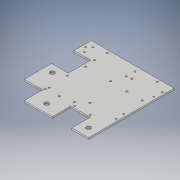
# Autodesk Inventor part: КВ33.044.002 - Дно платы
Saved by Autodesk Inventor 2019 (Build 230136000, 136)
## iProperties
Created: 2019-10-30
Part Number: КВ33.044.002 - Дно платы
Material: Типовые
Document SubType Name: Modeling
Designer: Петров Иван
Density: 1 g/cm^3
Appearance: По умолчанию
Mass: 56.5933 g
Surface Area: 408.613 cm^2
Volume: 56.5933 cm^3
Author: Петров Иван
Autodesk Inventor part; units mm, degrees
ref_plane "YZ Plane" through (0, 0, 0) normal (1, 0, 0) x (0, 1, 0)
ref_plane "XZ Plane" through (0, 0, 0) normal (0, 1, 0) x (-1, 0, 0)
ref_plane "XY Plane" through (0, 0, 0) normal (0, 0, 1) x (1, 0, 0)
sketch "Эскиз1" plane through (0, 0, 0) normal (0, 1, 0) x (-1, 0, 0)
  line L0 (-25, 35) -> (25, 35)
  line L1 (25, 35) -> (25, -35)
  line L2 (25, -35) -> (-25, -35)
  line L3 (-25, -35) -> (-25, 35)
  line L4 (-22.5, 32.5) -> (22.5, 32.5)
  line L5 (22.5, 31.5) -> (22.5, -31)
  line L6 (22.5, -32.5) -> (-22.5, -32.5)
  circle A0 centre (22.5, 32.5) radius 1.5
  circle A1 centre (22.5, -32.5) radius 1.5
  circle A2 centre (-22.5, -32.5) radius 1.5
  circle A3 centre (-22.5, 32.5) radius 1.5
  line L7 (-25, 35) -> (-23.7767, 33.2874) construction
  line L8 (-22.5, -31) -> (-22.5, 31)
  line L9 (23.7767, -33.2874) -> (25, -35) construction
  line L10 (25, -30.9585) -> (25, 35)
  line L11 (25, 35) -> (-25, 35)
  line L12 (25, 35) -> (25, -35)
  point P0 (0, 0)
  dimension "d6" = 3
  dimension "d0" = 50
  dimension "d2" = 45
  dimension "d4" = 3
  dimension "d5" = 3
  dimension "d7" = 3
  constraints: 26 end point, 4 coincident, 4 parallel, 4 point on circle, 3 centre point, 3 horizontal, 2 perpendicular, 2 point on line, 1 vertical alignment, 2 other
  measures "d0" distance of L1.end L2.end
  measures "d2" distance of L6.start L6.end
  measures "d4" diameter of A0
  measures "d5" diameter of A1
  measures "d7" diameter of A3
extrude "Выдавливание1" add sketch "Эскиз1" along normal blind 3 contours L0 L1 L2 L3 | L4 A0 L5 A1 L6 A2 L8 A3
sketch "Эскиз2" plane through (0, 3, 0) normal (0, 1, 0) x (1, 0, 0)
  line L0 (-25, -35) -> (25, -35) projected
  line L1 (-25, -35) -> (-28, -35)
  line L2 (-28, -35) -> (-28, 35)
  line L3 (-28, 35) -> (-25, 35)
  line L4 (-25, 35) -> (-25, -35)
  line L5 (-28, -35) -> (-58, -35)
  line L6 (-58, -35) -> (-58, 35)
  line L7 (-58, 35) -> (-28, 35)
  line L8 (-28, 35) -> (-28, -35)
  line L9 (-25, -35) -> (25, -35)
  line L10 (25, -35) -> (25, -38)
  line L11 (25, -38) -> (-25, -38)
  line L12 (-25, -38) -> (-25, -35)
  line L13 (-25, -38) -> (25, -38)
  line L14 (25, -38) -> (25, -68)
  line L15 (25, -68) -> (-25, -68)
  line L16 (-25, -68) -> (-25, -38)
  line L17 (-25, -68) -> (0, -68)
  line L18 (0, -53) -> (-25, -53)
  line L19 (-25, -53) -> (-25, -68)
  circle A0 centre (0, -53) radius 4
  line L20 (-58, 0) -> (-43, 0)
  circle A1 centre (-43, 0) radius 4
  point P0 (0, 0)
  dimension "d18" = 3
  dimension "d19" = 70
  dimension "d20" = 30
  dimension "d21" = 70
  dimension "d22" = 50
  dimension "d23" = 3
  dimension "d24" = 50
  dimension "d25" = 30
  dimension "d26" = 25
  dimension "d27" = 15
  dimension "d28" = 8
  dimension "d29" = 15
  dimension "d30" = 8
  constraints: 40 end point, 9 parallel, 6 horizontal, 4 perpendicular, 2 centre point, 2 coincident, 1 midpoint
  measures "d18" distance of L2.end L3.end
  measures "d19" distance of L1.end L2.end
  measures "d20" distance of L6.end L7.end
  measures "d21" distance of L5.end L6.end
  measures "d22" distance of L10.end L11.end
  measures "d23" distance of L9.end L10.end
  measures "d24" distance of L14.end L15.end
  measures "d25" distance of L13.end L14.end
  measures "d26" distance of L18.end L18.start
  measures "d27" distance of L18.start L17.end
  measures "d28" diameter of A0
  measures "d29" distance of L20.start L20.end
  measures "d30" diameter of A1
extrude "Выдавливание2" add sketch "Эскиз2" against normal blind 3
sketch "Эскиз3" plane through (0, 3, 0) normal (0, 1, 0) x (1, 0, 0)
  line L0 (-58, -35) -> (-25, -35) projected
  line L1 (-25, -35) -> (25, -35)
  line L2 (25, 35) -> (25, -68) projected
  line L3 (25, -35) -> (75, -35)
  line L4 (75, -35) -> (75, 35)
  line L5 (75, 35) -> (25, 35)
  line L6 (25, 35) -> (25, -35)
  point P0 (0, 0)
  dimension "d33" = 50
  constraints: 10 end point, 2 horizontal, 2 parallel, 1 perpendicular, 1 point on line
  measures "d33" distance of L5.end L4.end
extrude "Выдавливание3" add sketch "Эскиз3" against normal blind 3
move faces "Перенос1" translate (0, 0, -50) faces at (30.6667, 2, -35)
move faces "Перенос2" translate (15, 0, 0) faces at (75, 2, -5)
sketch "Эскиз5" plane through (0, 3, 0) normal (0, 1, 0) x (1, 0, 0)
  line L0 (35.0105, -28.2915) -> (88.3505, -28.2915)
  line L1 (88.3505, -28.2915) -> (88.3505, 70.7685)
  line L2 (88.3505, 70.7685) -> (87.0805, 70.7685)
  line L3 (87.0805, 70.7685) -> (84.5405, 73.3085)
  line L4 (84.5405, 73.3085) -> (50.2505, 73.3085)
  line L5 (50.2505, 73.3085) -> (47.7105, 70.7685)
  line L6 (47.7105, 70.7685) -> (37.5505, 70.7685)
  line L7 (37.5505, 70.7685) -> (35.0105, 68.2285)
  line L8 (35.0105, 68.2285) -> (35.0105, -28.2915)
  circle A0 centre (62.9505, 35.3355) radius 0.544
  circle A1 centre (40.0905, 68.2285) radius 0.544
  circle A2 centre (52.7905, 37.7485) radius 1.636
  circle A3 centre (85.8105, -14.3215) radius 1.636
  circle A4 centre (42.6305, 68.2285) radius 0.544
  circle A5 centre (85.8105, 68.2285) radius 1.636
  circle A6 centre (37.5505, 25.0485) radius 0.544
  circle A7 centre (45.1705, 68.2285) radius 0.544
  circle A8 centre (37.5505, 17.4285) radius 0.544
  circle A9 centre (57.8705, 35.3355) radius 0.544
  circle A10 centre (47.7105, 68.2285) radius 0.544
  circle A11 centre (60.4105, 37.8755) radius 0.544
  circle A12 centre (37.5505, 3.2045) radius 0.544
  circle A13 centre (50.2505, 68.2285) radius 0.544
  circle A14 centre (37.5505, -4.4155) radius 0.544
  circle A15 centre (37.5505, 35.2085) radius 0.544
  circle A16 centre (52.7905, 68.2285) radius 0.544
  circle A17 centre (37.5505, 27.5885) radius 0.544
  circle A18 centre (85.8105, 17.4285) radius 0.544
  circle A19 centre (55.3305, 68.2285) radius 0.544
  circle A20 centre (80.0447, -22.6019) radius 1.687
  circle A21 centre (37.5505, 13.3645) radius 0.544
  circle A22 centre (57.8705, 68.2285) radius 0.544
  circle A23 centre (37.5505, 5.7445) radius 0.544
  circle A24 centre (85.8105, 35.2085) radius 0.544
  circle A25 centre (60.4105, 68.2285) radius 0.544
  circle A26 centre (85.8105, 4.7285) radius 0.544
  circle A27 centre (85.8105, 7.2685) radius 0.544
  circle A28 centre (62.9505, 68.2285) radius 0.544
  circle A29 centre (85.8105, 14.8885) radius 0.544
  circle A30 centre (37.5505, 45.3685) radius 0.544
  circle A31 centre (65.4905, 68.2285) radius 0.544
  circle A32 centre (85.8105, 22.5085) radius 0.544
  circle A33 centre (85.8105, 25.0485) radius 0.544
  circle A34 centre (68.0305, 68.2285) radius 0.544
  circle A35 centre (85.8105, 32.6685) radius 0.544
  circle A36 centre (85.8105, 58.0685) radius 0.544
  circle A37 centre (70.5705, 68.2285) radius 0.544
  circle A38 centre (37.5505, 58.0685) radius 0.544
  circle A39 centre (37.5505, 55.5285) radius 0.544
  circle A40 centre (73.1105, 68.2285) radius 0.544
  circle A41 centre (37.5505, 47.9085) radius 0.544
  circle A42 centre (51.5205, -21.7637) radius 0.5185
  circle A43 centre (75.6505, 68.2285) radius 0.544
  circle A44 centre (85.8105, 45.3685) radius 0.544
  circle A45 centre (85.8105, 47.9085) radius 0.544
  circle A46 centre (78.1905, 68.2285) radius 0.544
  circle A47 centre (85.8105, 55.5285) radius 0.544
  circle A48 centre (80.7305, 68.2285) radius 0.544
  circle A49 centre (51.5205, -19.7571) radius 0.5185
  circle A50 centre (49.0005, -21.7637) radius 0.5185
  circle A51 centre (37.5505, 68.2285) radius 0.544
  circle A52 centre (76.2855, 8.5385) radius 0.341
  circle A53 centre (57.8705, -12.5435) radius 0.341
  circle A54 centre (43.3925, -7.4635) radius 0.544
  circle A55 centre (43.3925, -10.0035) radius 0.544
  circle A56 centre (71.2055, 8.5385) radius 0.341
  circle A57 centre (73.1105, -11.7815) radius 0.239
  circle A58 centre (47.5835, 2.5695) radius 0.239
  circle A59 centre (67.6495, 32.2875) radius 0.239
  circle A60 centre (65.8715, 32.5415) radius 0.239
  circle A61 centre (57.4895, 16.2855) radius 0.239
  circle A62 centre (54.2129, 34.8529) radius 0.239
  circle A63 centre (49.2345, 55.1475) radius 0.239
  circle A64 centre (83.3975, 2.0615) radius 0.239
  circle A65 centre (74.3805, -25.7515) radius 0.239
  circle A66 centre (66.1255, -25.7515) radius 0.239
  circle A67 centre (66.1255, -23.8465) radius 0.239
  circle A68 centre (66.1255, -21.9415) radius 0.239
  circle A69 centre (46.8215, -4.6695) radius 0.239
  circle A70 centre (53.8065, -8.9875) radius 0.239
  circle A71 centre (74.3805, -20.0365) radius 0.239
  circle A72 centre (74.3805, -23.8465) radius 0.239
  circle A73 centre (54.9495, 16.9205) radius 0.239
  circle A74 centre (67.1415, 9.9355) radius 0.239
  circle A75 centre (56.9815, 32.5415) radius 0.239
  circle A76 centre (62.3155, -9.8765) radius 0.239
  circle A77 centre (74.3805, -14.7025) radius 0.239
  circle A78 centre (52.6381, 44.2001) radius 0.239
  circle A79 centre (49.7425, 59.3385) radius 0.239
  circle A80 centre (54.6955, 4.3475) radius 0.239
  circle A81 centre (47.9645, 15.5235) radius 0.239
  circle A82 centre (46.9485, 30.0015) radius 0.239
  circle A83 centre (46.6945, -9.7495) radius 0.239
  circle A84 centre (67.1415, 12.4755) radius 0.239
  circle A85 centre (67.9035, 29.7475) radius 0.239
  circle A86 centre (45.0435, -3.7805) radius 0.239
  circle A87 centre (66.2525, -15.0835) radius 0.239
  circle A88 centre (82.6609, 20.0955) radius 0.239
  circle A89 centre (61.2995, 43.3365) radius 0.239
  circle A90 centre (64.4745, 51.5915) radius 0.239
  circle A91 centre (70.2911, 48.4165) radius 0.239
  circle A92 centre (63.7125, 9.4275) radius 0.239
  circle A93 centre (68.1575, -10.0035) radius 0.239
  circle A94 centre (36.9155, 37.8755) radius 0.239
  circle A95 centre (55.9655, -11.0195) radius 0.239
  circle A96 centre (56.2449, 42.0665) radius 0.239
  circle A97 centre (56.2195, 51.7185) radius 0.239
  circle A98 centre (78.9525, 3.2045) radius 0.239
  circle A99 centre (79.5875, 50.3215) radius 0.239
  circle A100 centre (42.5035, -0.0975) radius 0.239
  circle A101 centre (48.3455, 17.8095) radius 0.239
  circle A102 centre (49.4885, 17.1745) radius 0.239
  circle A103 centre (41.6145, 31.7795) radius 0.239
  circle A104 centre (49.7171, 47.6799) radius 0.239
  circle A105 centre (70.6975, 45.7495) radius 0.239
  circle A106 centre (78.1905, 6.3795) radius 0.239
  circle A107 centre (48.9805, 20.9845) radius 0.239
  circle A108 centre (45.6785, 20.4765) radius 0.239
  circle A109 centre (45.0435, 24.9215) radius 0.239
  circle A110 centre (46.3135, 23.6515) radius 0.239
  circle A111 centre (45.1705, 23.0165) radius 0.239
  circle A112 centre (49.2345, 53.1155) radius 0.239
  circle A113 centre (78.2159, 22.3815) radius 0.239
  circle A114 centre (79.5875, 52.7345) radius 0.239
  circle A115 centre (65.3635, 16.2855) radius 0.239
  circle A116 centre (46.3135, 26.3185) radius 0.239
  circle A117 centre (51.6475, 3.2045) radius 0.239
  circle A118 centre (53.1715, 12.0945) radius 0.239
  circle A119 centre (78.0635, 20.9591) radius 0.239
  circle A120 centre (77.4285, 45.6225) radius 0.239
  circle A121 centre (59.5215, 12.7295) radius 0.239
  circle A122 centre (70.4435, 44.3525) radius 0.239
  circle A123 centre (49.9965, -6.3205) radius 0.239
  circle A124 centre (51.9015, 12.3485) radius 0.239
  circle A125 centre (66.8875, 30.7635) radius 0.239
  circle A126 centre (62.9505, 16.9205) radius 0.239
  circle A127 centre (40.9795, 36.9865) radius 0.239
  circle A128 centre (58.6325, 27.4615) radius 0.239
  circle A129 centre (59.5215, 11.4595) radius 0.239
  circle A130 centre (56.4735, 27.4615) radius 0.239
  circle A131 centre (76.7935, 21.1115) radius 0.239
  circle A132 centre (69.6815, 30.7635) radius 0.239
  circle A133 centre (70.1895, -2.5105) radius 0.239
  circle A134 centre (41.2335, 22.3815) radius 0.239
  circle A135 centre (69.1735, 43.7175) radius 0.239
  circle A136 centre (40.9795, 38.5105) radius 0.239
  circle A137 centre (63.2045, 12.6025) radius 0.239
  circle A138 centre (40.9795, 21.1115) radius 0.239
  circle A139 centre (54.8225, 11.3325) radius 0.239
  circle A140 centre (50.3775, 2.3155) radius 0.239
  circle A141 centre (48.0915, 26.3185) radius 0.239
  circle A142 centre (79.7145, 20.7305) radius 0.239
  circle A143 centre (64.2205, 11.5865) radius 0.239
  circle A144 centre (78.1905, 47.5275) radius 0.239
  circle A145 centre (71.4595, 47.0195) radius 0.239
  circle A146 centre (47.8375, 22.1275) radius 0.239
  circle A147 centre (44.1545, 24.0325) radius 0.239
  circle A148 centre (44.1545, 25.8105) radius 0.239
  circle A149 centre (44.7895, 21.3655) radius 0.239
  circle A150 centre (46.0595, 22.1275) radius 0.239
  circle A151 centre (65.7445, -4.2885) radius 0.239
  circle A152 centre (49.3615, 50.4485) radius 0.239
  circle A153 centre (41.6145, 51.8455) radius 0.239
  circle A154 centre (41.6145, 2.1885) radius 0.239
  circle A155 centre (47.4565, 18.6985) radius 0.239
  circle A156 centre (46.5675, 19.5875) radius 0.239
  circle A157 centre (76.6665, -1.7485) radius 0.239
  circle A158 centre (80.0701, 18.5715) radius 0.239
  circle A159 centre (61.0455, 51.7185) radius 0.239
  circle A160 centre (80.9845, -4.2885) radius 0.239
  circle A161 centre (68.3353, 34.7259) radius 0.239
  circle A162 centre (71.8405, 71.5305) radius 0.239
  circle A163 centre (37.5505, -6.1935) radius 0.239
  circle A164 centre (49.9965, 13.7963) radius 0.239
  circle A165 centre (60.6645, 49.6865) radius 0.239
  circle A166 centre (56.6005, 71.5305) radius 0.239
  circle A167 centre (64.4745, 42.0665) radius 0.239
  circle A168 centre (59.5215, -10.0035) radius 0.239
  circle A169 centre (84.9215, -2.5105) radius 0.239
  circle A170 centre (61.8075, -4.1615) radius 0.239
  circle A171 centre (60.5375, 32.5415) radius 0.239
  circle A172 centre (59.3945, -16.0995) radius 0.239
  circle A173 centre (51.1395, -11.0195) radius 0.239
  circle A174 centre (64.0935, -2.7645) radius 0.239
  circle A175 centre (40.5477, 49.2039) radius 0.239
  circle A176 centre (61.0455, 16.4125) radius 0.239
  circle A177 centre (59.1151, 10.0625) radius 0.239
  circle A178 centre (67.3955, 59.4655) radius 0.239
  circle A179 centre (76.6665, -3.6535) radius 0.239
  circle A180 centre (72.3485, 4.3475) radius 0.239
  circle A181 centre (60.4105, 27.5885) radius 0.239
  circle A182 centre (68.3353, 40.7203) radius 0.239
  circle A183 centre (59.6485, 16.7935) radius 0.239
  circle A184 centre (49.4885, 26.9535) radius 0.239
  circle A185 centre (72.4755, -19.4015) radius 0.239
  circle A186 centre (52.9175, -12.9245) radius 0.239
  circle A187 centre (60.2835, -0.2245) radius 0.239
  circle A188 centre (71.9675, -4.4155) radius 0.239
  circle A189 centre (59.1405, -19.4015) radius 0.239
  circle A190 centre (66.1255, -20.0365) radius 0.239
  circle A191 centre (68.6655, -19.4015) radius 0.239
  circle A192 centre (74.3805, -21.9415) radius 0.239
  circle A193 centre (74.1265, 3.9665) radius 0.239
  circle A194 centre (54.1875, 28.1981) radius 0.239
  circle A195 centre (61.6805, 28.7315) radius 0.239
  circle A196 centre (51.6475, 15.3965) radius 0.239
  circle A197 centre (68.7925, 31.6525) radius 0.239
  circle A198 centre (59.2675, 32.0335) radius 0.239
  circle A199 centre (46.7453, -11.3243) radius 0.239
  circle A200 centre (45.6785, -18.6395) radius 0.239
  circle A201 centre (40.8525, -12.5435) radius 0.544
  circle A202 centre (40.8525, -10.0035) radius 0.544
  circle A203 centre (40.8525, -7.4635) radius 0.544
  circle A204 centre (57.8705, -7.4635) radius 0.341
  circle A205 centre (37.5505, 65.6885) radius 0.544
  circle A206 centre (43.3925, -12.5435) radius 0.544
  circle A207 centre (49.0005, -19.7571) radius 0.5185
  circle A208 centre (80.7305, 65.6885) radius 0.544
  circle A209 centre (78.1905, 65.6885) radius 0.544
  circle A210 centre (85.8105, 52.9885) radius 0.544
  circle A211 centre (85.8105, 50.4485) radius 0.544
  circle A212 centre (75.6505, 65.6885) radius 0.544
  circle A213 centre (56.2703, -24.4815) radius 1.141
  circle A214 centre (44.2505, -24.4815) radius 1.141
  circle A215 centre (73.1105, 65.6885) radius 0.544
  circle A216 centre (37.5505, 50.4485) radius 0.544
  circle A217 centre (37.5505, 52.9885) radius 0.544
  circle A218 centre (70.5705, 65.6885) radius 0.544
  circle A219 centre (85.8105, 63.1485) radius 0.544
  circle A220 centre (85.8105, 60.6085) radius 0.544
  circle A221 centre (68.0305, 65.6885) radius 0.544
  circle A222 centre (85.8105, 30.1285) radius 0.544
  circle A223 centre (85.8105, 27.5885) radius 0.544
  circle A224 centre (65.4905, 65.6885) radius 0.544
  circle A225 centre (37.5505, 40.2885) radius 0.544
  circle A226 centre (37.5505, 42.8285) radius 0.544
  circle A227 centre (62.9505, 65.6885) radius 0.544
  circle A228 centre (85.8105, 12.3485) radius 0.544
  circle A229 centre (85.8105, 9.8085) radius 0.544
  circle A230 centre (60.4105, 65.6885) radius 0.544
  circle A231 centre (85.8105, 40.2885) radius 0.544
  circle A232 centre (85.8105, 37.7485) radius 0.544
  circle A233 centre (57.8705, 65.6885) radius 0.544
  circle A234 centre (37.5505, 8.2845) radius 0.544
  circle A235 centre (37.5505, 10.8245) radius 0.544
  circle A236 centre (55.3305, 65.6885) radius 0.544
  circle A237 centre (80.0447, -16.6075) radius 1.687
  circle A238 centre (85.0485, -19.6047) radius 1.687
  circle A239 centre (52.7905, 65.6885) radius 0.544
  circle A240 centre (37.5505, 30.1285) radius 0.544
  circle A241 centre (37.5505, 32.6685) radius 0.544
  circle A242 centre (50.2505, 65.6885) radius 0.544
  circle A243 centre (37.5505, -1.8755) radius 0.544
  circle A244 centre (37.5505, 0.6645) radius 0.544
  circle A245 centre (47.7105, 65.6885) radius 0.544
  circle A246 centre (60.4105, 35.3355) radius 0.544
  circle A247 centre (57.8705, 37.8755) radius 0.544
  circle A248 centre (45.1705, 65.6885) radius 0.544
  circle A249 centre (37.5505, 19.9685) radius 0.544
  circle A250 centre (37.5505, 22.5085) radius 0.544
  circle A251 centre (42.6305, 65.6885) radius 0.544
  circle A252 centre (37.5505, -13.0515) radius 1.636
  circle A253 centre (37.5505, 61.8785) radius 1.636
  circle A254 centre (40.0905, 65.6885) radius 0.544
  circle A255 centre (80.7305, 37.7485) radius 1.636
  circle A256 centre (62.9505, 37.8755) radius 0.544
  point P0 (0, 0)
  point P1 (61.6805, -28.2915)
  constraints: 257 centre point, 18 end point
extrude "Выдавливание5" cut sketch "Эскиз5" against normal blind 10 contours A2 | A3 | A5 | A252 | A253 | A255
sketch "Эскиз6" plane through (0, 3, 0) normal (0, 1, 0) x (1, 0, 0)
  line L0 (-25, -35) -> (25, -35)
  line L1 (25, -35) -> (25, 35)
  line L2 (25, 35) -> (-25, 35)
  line L3 (-25, 35) -> (-25, -35)
  line L4 (-25, -35) -> (25, 35) construction
  line L5 (25, -35) -> (-25, 35) construction
  point P0 (0, 0)
  dimension "d46" = 50
  dimension "d47" = 70
  constraints: 12 end point, 2 midpoint, 2 parallel, 1 horizontal, 1 perpendicular
  measures "d46" distance of L2.end L1.end
  measures "d47" distance of L1.end L0.end
extrude "Выдавливание6" add sketch "Эскиз6" against normal blind 3
sketch "Эскиз7" plane through (0, 3, 0) normal (0, 1, 0) x (1, 0, 0)
  line L0 (-25, 41.6193) -> (25, 41.6193)
  line L1 (25, 41.6193) -> (25, -28.3807)
  line L2 (25, -28.3807) -> (-25, -28.3807)
  line L3 (-25, -28.3807) -> (-25, 41.6193)
  line L4 (-22.5, 39.1193) -> (22.5, 39.1193)
  line L5 (22.5, 38.1193) -> (22.5, -24.3807)
  line L6 (22.5, -25.8807) -> (-22.5, -25.8807)
  circle A0 centre (22.5, 39.1193) radius 1.5
  circle A1 centre (22.5, -25.8807) radius 1.5
  circle A2 centre (-22.5, -25.8807) radius 1.5
  circle A3 centre (-22.5, 39.1193) radius 1.5
  line L7 (-25, 41.6193) -> (-23.7767, 39.9067) construction
  line L8 (-22.5, -24.3807) -> (-22.5, 37.6193)
  line L9 (23.7767, -26.6681) -> (25, -28.3807) construction
  line L10 (25, -24.3391) -> (25, 41.6193)
  line L11 (25, 41.6193) -> (-25, 41.6193)
  line L12 (25, 41.6193) -> (25, -28.3807)
  point P0 (0, 0)
  point P1 (0, 6.6193)
  dimension "d54" = 3
  dimension "d50" = 50
  dimension "d51" = 45
  dimension "d52" = 3
  dimension "d53" = 3
  dimension "d55" = 3
  constraints: 26 end point, 4 coincident, 4 parallel, 4 point on circle, 3 centre point, 3 horizontal, 2 perpendicular, 2 point on line, 1 vertical alignment, 2 other
  measures "d50" distance of L1.end L2.end
  measures "d51" distance of L6.start L6.end
  measures "d52" diameter of A0
  measures "d53" diameter of A1
  measures "d55" diameter of A3
extrude "Выдавливание7" cut sketch "Эскиз7" against normal blind 3 contours A3 | A0 | A2 | A1
sketch "Эскиз8" plane through (0, 3, 0) normal (0, 1, 0) x (1, 0, 0)
  circle A0 centre (-46.0635, 75.8151) radius 1.5
  circle A1 centre (-46.0635, 60.8151) radius 1.5
  circle A2 centre (28.9365, 60.8151) radius 1.5
  circle A3 centre (28.9365, 75.8151) radius 1.5
  point P0 (0, 0)
  point P1 (-16.0911, 67.0392)
  dimension "d60" = 3
  dimension "d61" = 3
  dimension "d62" = 3
  dimension "d63" = 3
  dimension "d64" = 15
  dimension "d65" = 75
  dimension "d68" = 75
  constraints: 4 centre point
  measures "d60" diameter of A0
  measures "d61" diameter of A1
  measures "d62" diameter of A2
  measures "d63" diameter of A3
  measures "d64" distance of A2.centre A3.centre
  measures "d65" distance of A0.centre A3.centre
  measures "d68" distance of A2.centre A1.centre
extrude "Выдавливание8" cut sketch "Эскиз8" against normal blind 3
sketch "Эскиз9" plane through (0, 3, 0) normal (0, 1, 0) x (1, 0, 0)
  line L0 (-58, -35) -> (-58, 85) projected
  line L1 (-58, 13.7892) -> (-28, 13.7892)
  line L2 (-28, 13.7892) -> (-28, 53.7892)
  line L3 (-28, 53.7892) -> (-58, 53.7892)
  line L4 (-58, 53.7892) -> (-58, 13.7892)
  point P0 (0, 0)
  dimension "d69" = 30
  dimension "d70" = 40
  constraints: 8 end point, 2 parallel, 1 horizontal, 1 perpendicular, 1 point on line
  measures "d69" distance of L3.end L2.end
  measures "d70" distance of L2.end L1.end
extrude "Выдавливание9" cut sketch "Эскиз9" against normal blind 3
sketch "Эскиз10" plane through (0, 3, 0) normal (0, 1, 0) x (1, 0, 0)
  line L0 (90, 85) -> (90, -35) projected
  line L1 (90, -35) -> (60, -35)
  line L2 (60, -35) -> (60, -68)
  line L3 (60, -68) -> (90, -68)
  line L4 (90, -68) -> (90, -35)
  circle A0 centre (75, -53) radius 4
  point P0 (0, 0)
  dimension "d73" = 30
  dimension "d74" = 33
  dimension "d75" = 8
  dimension "d109" = 15
  dimension "d110" = 15
  constraints: 8 end point, 2 parallel, 1 centre point, 1 horizontal, 1 perpendicular
  measures "d73" distance of L3.end L2.end
  measures "d74" distance of L2.end L1.end
  measures "d75" diameter of A0
  measures "d109" distance from line of L3 A0.centre
  measures "d110" distance from line of L2 A0.centre
extrude "Выдавливание10" add sketch "Эскиз10" against normal blind 3
sketch "Эскиз11" plane through (0, 3, 0) normal (0, 1, 0) x (1, 0, 0)
  line L0 (-58, -35) -> (-25, -35) projected
  line L1 (60, -35) -> (25, -35) projected
  line L2 (-25, -35) -> (25, -35)
  line L3 (0, -35) -> (0, -30)
  circle A0 centre (0, -30) radius 1.5
  line L4 (-28, 13.7892) -> (-28, 53.7892) projected
  circle A1 centre (-25, 8.7892) radius 1.5
  line L5 (-58, 53.7892) -> (-58, 85) projected
  line L6 (-58, 69.3946) -> (-53, 69.3946)
  circle A2 centre (-53, 69.3946) radius 1.5
  line L7 (-28, 53.7892) -> (-58, 53.7892) projected
  line L8 (-28, 53.7892) -> (-24.4645, 57.3247)
  line L9 (-28, 53.7892) -> (-23, 53.7892) construction
  circle A3 centre (-24.4645, 57.3247) radius 1.5
  line L10 (-24.4645, 57.3247) -> (-24.4645, 85)
  line L11 (-58, 85) -> (90, 85) projected
  line L12 (-24.4645, 85) -> (-24.4645, 80)
  circle A4 centre (-24.4645, 80) radius 1.5
  line L13 (65, 85) -> (65, 80)
  circle A5 centre (65, 80) radius 1.5
  line L14 (90, -68) -> (90, 85) projected
  line L15 (90, 85) -> (90, -68) projected
  line L16 (90, 53.7892) -> (85, 53.7892)
  circle A6 centre (85, 53.7892) radius 1.5
  line L17 (60, -35) -> (90, -35)
  line L18 (90, 0) -> (85, 0)
  circle A7 centre (85, 0) radius 1.5
  line L19 (25, -35) -> (25, -68) projected
  line L20 (25, -35) -> (28.5355, -31.4645)
  line L21 (25, -35) -> (30, -35) construction
  circle A8 centre (28.5355, -31.4645) radius 1.5
  line L22 (60, -35) -> (56.4645, -31.4645)
  line L23 (60, -35) -> (65, -35) construction
  circle A9 centre (56.4645, -31.4645) radius 1.5
  line L24 (-24, -35) -> (-24, -32)
  circle A10 centre (-24, -32) radius 1.5
  line L25 (-28, 13.7892) -> (-58, 13.7892) projected
  line L26 (-58, 13.7892) -> (-58, -35) projected
  point P0 (0, 0)
  dimension "d78" = 5
  dimension "d79" = 3
  dimension "d81" = 3
  dimension "d82" = 5
  dimension "d83" = 3
  dimension "d84" = 5
  dimension "d85" = 45
  dimension "d86" = 3
  dimension "d87" = 5
  dimension "d88" = 3
  dimension "d89" = 5
  dimension "d90" = 3
  dimension "d91" = 25
  dimension "d92" = 5
  dimension "d93" = 3
  dimension "d94" = 5
  dimension "d95" = 3
  dimension "d96" = 5
  dimension "d97" = 45
  dimension "d98" = 3
  dimension "d99" = 5
  dimension "d100" = 135
  dimension "d101" = 3
  dimension "d102" = 3
  dimension "d103" = 3
  dimension "d106" = 5
  dimension "d107" = 3
  dimension "d108" = 34
  constraints: 32 end point, 11 centre point, 10 coincident, 7 point on line, 4 horizontal, 4 vertical, 3 equal length, 3 perpendicular, 2 midpoint, 1 collinear
  measures "d78" distance of L3.start L3.end
  measures "d79" diameter of A0
  measures "d81" diameter of A1
  measures "d82" distance of L6.start L6.end
  measures "d83" diameter of A2
  measures "d84" distance of L4.end L8.end
  measures "d85" angle of L9 L8
  measures "d86" diameter of A3
  measures "d87" distance of L10.end L12.end
  measures "d88" diameter of A4
  measures "d89" distance of L13.start L13.end
  measures "d90" diameter of A5
  measures "d91" distance between parallel lines of L14 L13
  measures "d92" distance of L16.start L16.end
  measures "d93" diameter of A6
  measures "d94" distance of L18.start L18.end
  measures "d95" diameter of A7
  measures "d96" distance of L1.end L20.end
  measures "d97" angle of L21 L20
  measures "d98" diameter of A8
  measures "d99" distance of L1.start L22.end
  measures "d100" angle of L23 L22
  measures "d101" diameter of A9
  measures "d102" distance of L24.start L24.end
  measures "d103" diameter of A10
  measures "d106" distance from line of L25 A1.centre
  measures "d107" distance from line of A1.centre L4
  measures "d108" distance between parallel lines of L26 L24
extrude "Выдавливание11" cut sketch "Эскиз11" against normal blind 10 contours A3 L10 L8 | L8 L10 A3 | A4 L10 | L10 A4 | A0 | A1 | A2 | A5 | A6 | A7 | A8 | A9 | A10
